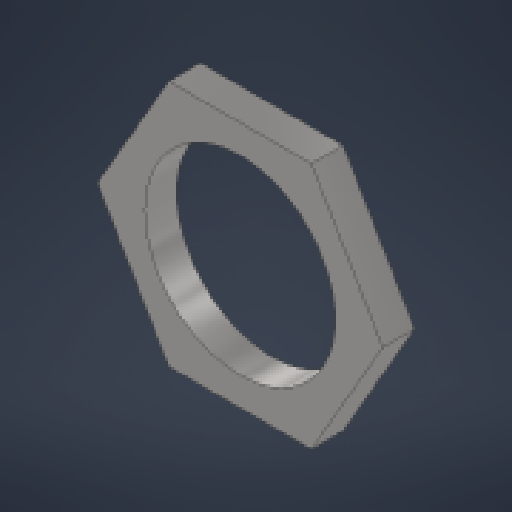
# Autodesk Inventor part: NKK_S1AL_mother
Saved by Autodesk Inventor 2024 (Build 280153000, 153)
## iProperties
Created: 2026-05-08
Part Number: NKK_S1AL_mother
Material: Stainless Steel
Document SubType Name: Modeling
Designer: schar
Density: 8 g/cm^3
Appearance: Semi-Polished
Author: schar
Autodesk Inventor part; units mm, degrees
ref_plane "YZ Plane" through (0, 0, 0) normal (1, 0, 0) x (0, 1, 0)
ref_plane "XZ Plane" through (0, 0, 0) normal (0, 1, 0) x (-1, 0, 0)
ref_plane "XY Plane" through (0, 0, 0) normal (0, 0, 1) x (1, 0, 0)
sketch "Sketch1" plane through (0, 0, 0) normal (0, 0, 1) x (1, 0, 0)
  circle A0 centre (-36.2, 0) radius 6 projected
  circle A1 centre (-36.2, 0) radius 6
  line L0 (-27.2099, 0) -> (-31.705, -7.7856)
  line L1 (-31.705, -7.7856) -> (-40.695, -7.7856)
  line L2 (-40.695, -7.7856) -> (-45.1901, 0)
  line L3 (-45.1901, 0) -> (-40.695, 7.7856)
  line L4 (-40.695, 7.7856) -> (-31.705, 7.7856)
  line L5 (-31.705, 7.7856) -> (-27.2099, 0)
  point P0 (0, 0)
  constraints: 12 end point, 2 coincident, 1 centre point, 1 concentric, 13 other
extrude "Extrusion1" add sketch "Sketch1" along normal blind 2
body "Solid1"
